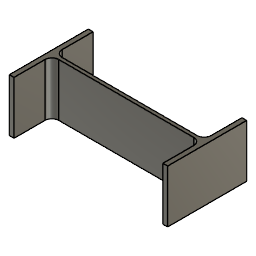
H-300×150×6×9 (Autodesk Fusion 360 design; units mm, degrees)
Autodesk Fusion 360 part; units mm, degrees
sketch "スケッチ1" plane through (0, 0, 0) normal (0, 0, 1) x (1, 0, 0)
  line L0 (0, 75) -> (0, -75)
  line L1 (300, -75) -> (300, 75)
  line L2 (291, -16.25) -> (291, -75)
  line L3 (9, -75) -> (9, -16.25)
  line L4 (0, -75) -> (9, -75)
  line L5 (291, -75) -> (300, -75)
  line L6 (278, 3.25) -> (22, 3.25)
  line L7 (22, -3.25) -> (278, -3.25)
  line L8 (9, 16.25) -> (9, 75)
  arc A0 (22, -3.25) -> (9, -16.25) centre (22, -16.25) ccw
  arc A1 (9, 16.25) -> (22, 3.25) centre (22, 16.25) ccw
  line L9 (9, 75) -> (0, 75)
  line L10 (291, 75) -> (291, 16.25)
  arc A2 (291, -16.25) -> (278, -3.25) centre (278, -16.25) ccw
  arc A3 (278, 3.25) -> (291, 16.25) centre (278, 16.25) ccw
  line L11 (300, 75) -> (291, 75)
extrude "押し出し1" add sketch "スケッチ1" along normal blind 100
